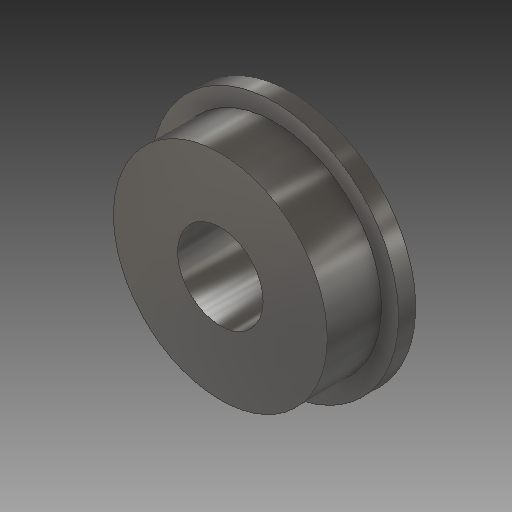
# Autodesk Inventor part: ベアリングフランジ付き0615.5t
Saved by Autodesk Inventor 2020 (Build 240168000, 168)
## iProperties
Created: 2018-11-20
Part Number: ベアリングフランジ付き0615.5t
Material: 鋼、高強度、低合金
Document SubType Name: Modeling
Designer: 雪村
Density: 7.85 g/cm^3
Appearance: 鋼 - つや出し
Mass: 6.40158 g
Surface Area: 7.57941 cm^2
Volume: 0.815488 cm^3
Author: 雪村
Autodesk Inventor part; units mm, degrees
ref_plane "YZ Plane" through (0, 0, 0) normal (1, 0, 0) x (0, 1, 0)
ref_plane "XZ Plane" through (0, 0, 0) normal (0, 1, 0) x (-1, 0, 0)
ref_plane "XY Plane" through (0, 0, 0) normal (0, 0, 1) x (1, 0, 0)
sketch "スケッチ1" plane through (0, 0, 0) normal (0, 0, 1) x (1, 0, 0)
  circle A0 centre (0, 0) radius 3
  circle A1 centre (0, 0) radius 7.5
  dimension "d0" = 6
  dimension "d1" = 15
  constraints: 2 centre point, 2 coincident
  measures "d0" diameter of A0
  measures "d1" diameter of A1
extrude "押し出し1" add sketch "スケッチ1" along normal blind 5
sketch "スケッチ2" plane through (0, 0, 0) normal (0, 0, -1) x (-1, 0, 0)
  circle A0 centre (0, 0) radius 8.7
  circle A1 centre (0, 0) radius 3 projected
  circle A2 centre (0, 0) radius 7.5 projected
  dimension "d7" = 1.2
  constraints: 1 centre point, 1 coincident
  measures "d7" radial gap between concentric circles of A2 A0
extrude "押し出し2" add sketch "スケッチ2" against normal blind 1.2 contours A0 | A2
